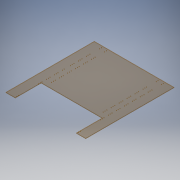
# Autodesk Inventor part: Top Aluminium Plate
Saved by Autodesk Inventor 2019.4 (Build 234330000, 330)
## iProperties
Created: 2019-12-08
Part Number: Top Aluminium Plate
Material: Polycarbonate, Smoke
Document SubType Name: Modeling
Designer: admin
Density: 1.2 g/cm^3
Appearance: Polycarbonate - Smoked
Mass: 1989.21 g
Surface Area: 8468.67 cm^2
Volume: 1657.67 cm^3
Author: admin
Autodesk Inventor part; units mm, degrees
ref_plane "YZ Plane" through (0, 0, 0) normal (1, 0, 0) x (0, 1, 0)
ref_plane "XZ Plane" through (0, 0, 0) normal (0, 1, 0) x (-1, 0, 0)
ref_plane "XY Plane" through (0, 0, 0) normal (0, 0, 1) x (1, 0, 0)
sketch "Sketch1" plane through (0, 0, 0) normal (0, 1, 0) x (-1, 0, 0)
  line L0 (323.8522, 485.9933) -> (327.8522, 485.9933) projected
  line L1 (327.8522, -234.0067) -> (327.8522, 485.9933) projected
  line L2 (-318.1478, -234.0067) -> (-322.1478, -234.0067) projected
  line L3 (-322.1478, -234.0067) -> (-322.1478, 485.9933) projected
  line L4 (327.8522, 485.9933) -> (-322.1478, 485.9933)
  line L5 (-322.1478, 485.9933) -> (-322.1478, -234.0067)
  line L6 (-322.1478, -234.0067) -> (327.8522, -234.0067)
  line L7 (327.8522, -234.0067) -> (327.8522, 485.9933)
  circle A0 centre (255.3522, -204.5067) radius 1.65 projected
  circle A1 centre (255.3522, -218.5067) radius 1.65 projected
  circle A2 centre (255.3522, 470.4933) radius 1.65 projected
  circle A3 centre (255.3522, 456.4933) radius 1.65 projected
  circle A4 centre (255.3522, 263.9913) radius 1.65 projected
  circle A5 centre (255.3522, 293.9913) radius 1.65 projected
  circle A6 centre (255.3522, 278.9913) radius 1.65 projected
  circle A7 centre (255.3522, -111.0087) radius 1.65 projected
  circle A8 centre (255.3522, -61.0087) radius 1.65 projected
  circle A9 centre (255.3522, -31.0087) radius 1.65 projected
  circle A10 centre (255.3522, 18.9913) radius 1.65 projected
  circle A11 centre (255.3522, 68.9913) radius 1.65 projected
  circle A12 centre (255.3522, 98.9913) radius 1.65 projected
  circle A13 centre (255.3522, 148.9913) radius 1.65 projected
  circle A14 centre (255.3522, 198.9913) radius 1.65 projected
  circle A15 centre (255.3522, 228.9913) radius 1.65 projected
  circle A16 centre (255.3522, 213.9913) radius 1.65 projected
  circle A17 centre (255.3522, 163.9913) radius 1.65 projected
  circle A18 centre (255.3522, 133.9913) radius 1.65 projected
  circle A19 centre (255.3522, 83.9913) radius 1.65 projected
  circle A20 centre (255.3522, 33.9913) radius 1.65 projected
  circle A21 centre (255.3522, 3.9913) radius 1.65 projected
  circle A22 centre (255.3522, -46.0087) radius 1.65 projected
  circle A23 centre (255.3522, -96.0087) radius 1.65 projected
  circle A24 centre (255.3522, -126.0087) radius 1.65 projected
  line L8 (251.8522, -234.0067) -> (251.8522, 485.9933) projected
  line L9 (251.8522, 485.9933) -> (258.8522, 485.9933) projected
  line L10 (258.8522, 485.9933) -> (258.8522, -234.0067) projected
  line L11 (258.8522, -234.0067) -> (251.8522, -234.0067) projected
  circle A25 centre (213.3522, -218.0067) radius 1.65 projected
  circle A26 centre (213.3522, -203.0067) radius 1.65 projected
  circle A27 centre (213.3522, 228.9913) radius 1.65 projected
  circle A28 centre (213.3522, 213.9913) radius 1.65 projected
  circle A29 centre (213.3522, 163.9913) radius 1.65 projected
  circle A30 centre (213.3522, 133.9913) radius 1.65 projected
  circle A31 centre (213.3522, 83.9913) radius 1.65 projected
  circle A32 centre (213.3522, 33.9913) radius 1.65 projected
  circle A33 centre (213.3522, 3.9913) radius 1.65 projected
  circle A34 centre (213.3522, -46.0087) radius 1.65 projected
  circle A35 centre (213.3522, -96.0087) radius 1.65 projected
  circle A36 centre (213.3522, -111.0087) radius 1.65 projected
  circle A37 centre (213.3522, -126.0087) radius 1.65 projected
  circle A38 centre (213.3522, -61.0087) radius 1.65 projected
  circle A39 centre (213.3522, -31.0087) radius 1.65 projected
  circle A40 centre (213.3522, 18.9913) radius 1.65 projected
  circle A41 centre (213.3522, 68.9913) radius 1.65 projected
  circle A42 centre (213.3522, 98.9913) radius 1.65 projected
  circle A43 centre (213.3522, 148.9913) radius 1.65 projected
  circle A44 centre (213.3522, 198.9913) radius 1.65 projected
  line L12 (209.8522, 274.709) -> (216.8522, 274.709) projected
  line L13 (216.8522, -234.0067) -> (216.8522, 274.709) projected
  line L14 (216.8522, -234.0067) -> (209.8522, -234.0067) projected
  line L15 (209.8522, -234.0067) -> (209.8522, 274.709) projected
  circle A45 centre (-249.6478, -204.5067) radius 1.65 projected
  circle A46 centre (-249.6478, -218.5067) radius 1.65 projected
  circle A47 centre (-249.6478, 470.4933) radius 1.65 projected
  circle A48 centre (-249.6478, 456.4933) radius 1.65 projected
  circle A49 centre (-249.6478, 263.9913) radius 1.65 projected
  circle A50 centre (-249.6478, 293.9913) radius 1.65 projected
  circle A51 centre (-249.6478, 278.9913) radius 1.65 projected
  circle A52 centre (-249.6478, -111.0087) radius 1.65 projected
  circle A53 centre (-249.6478, -61.0087) radius 1.65 projected
  circle A54 centre (-249.6478, -31.0087) radius 1.65 projected
  circle A55 centre (-249.6478, 18.9913) radius 1.65 projected
  circle A56 centre (-249.6478, 68.9913) radius 1.65 projected
  circle A57 centre (-249.6478, 98.9913) radius 1.65 projected
  circle A58 centre (-249.6478, 148.9913) radius 1.65 projected
  circle A59 centre (-249.6478, 198.9913) radius 1.65 projected
  circle A60 centre (-249.6478, 228.9913) radius 1.65 projected
  circle A61 centre (-249.6478, 213.9913) radius 1.65 projected
  circle A62 centre (-249.6478, 163.9913) radius 1.65 projected
  circle A63 centre (-249.6478, 133.9913) radius 1.65 projected
  circle A64 centre (-249.6478, 83.9913) radius 1.65 projected
  circle A65 centre (-249.6478, 33.9913) radius 1.65 projected
  circle A66 centre (-249.6478, 3.9913) radius 1.65 projected
  circle A67 centre (-249.6478, -46.0087) radius 1.65 projected
  circle A68 centre (-249.6478, -96.0087) radius 1.65 projected
  circle A69 centre (-249.6478, -126.0087) radius 1.65 projected
  line L16 (-246.1478, -234.0067) -> (-246.1478, 485.9933) projected
  line L17 (-253.1478, -234.0067) -> (-246.1478, -234.0067) projected
  line L18 (-253.1478, 485.9933) -> (-253.1478, -234.0067) projected
  line L19 (-246.1478, 485.9933) -> (-253.1478, 485.9933) projected
  circle A70 centre (-207.6478, -218.0067) radius 1.65 projected
  circle A71 centre (-207.6478, -203.0067) radius 1.65 projected
  circle A72 centre (-207.6478, 228.9913) radius 1.65 projected
  circle A73 centre (-207.6478, 213.9913) radius 1.65 projected
  circle A74 centre (-207.6478, 163.9913) radius 1.65 projected
  circle A75 centre (-207.6478, 133.9913) radius 1.65 projected
  circle A76 centre (-207.6478, 83.9913) radius 1.65 projected
  circle A77 centre (-207.6478, 33.9913) radius 1.65 projected
  circle A78 centre (-207.6478, 3.9913) radius 1.65 projected
  circle A79 centre (-207.6478, -46.0087) radius 1.65 projected
  circle A80 centre (-207.6478, -96.0087) radius 1.65 projected
  circle A81 centre (-207.6478, -111.0087) radius 1.65 projected
  circle A82 centre (-207.6478, -126.0087) radius 1.65 projected
  circle A83 centre (-207.6478, -61.0087) radius 1.65 projected
  circle A84 centre (-207.6478, -31.0087) radius 1.65 projected
  circle A85 centre (-207.6478, 18.9913) radius 1.65 projected
  circle A86 centre (-207.6478, 68.9913) radius 1.65 projected
  circle A87 centre (-207.6478, 98.9913) radius 1.65 projected
  circle A88 centre (-207.6478, 148.9913) radius 1.65 projected
  circle A89 centre (-207.6478, 198.9913) radius 1.65 projected
  line L20 (-204.1478, 274.709) -> (-211.1478, 274.709) projected
  line L21 (-204.1478, -234.0067) -> (-204.1478, 274.709) projected
  line L22 (-211.1478, -234.0067) -> (-204.1478, -234.0067) projected
  line L23 (-211.1478, -234.0067) -> (-211.1478, 274.709) projected
  constraints: 6 end point, 2 horizontal, 1 parallel, 1 perpendicular, 3 other
extrude "Extrusion1" add sketch "Sketch1" along normal blind 4 contours L0 L1 L6 L10 L4 | L10 L6 L8 L4 | L8 L6 L13 L12 L15 L21 L20 L23 L16 L4 | L16 L6 L18 L4 | L18 L6 L2 L3 L4 | L6 L15 L12 L13 | L23 L20 L21 L6 | A0 | A1 | A2 | A3 | A4 | A5 | A6 | A7 | A8 | A9 | A10 | A11 | A12 | A13 | A14 | A15 | A16 | A17 | A18 | A19 | A20 | A21 | A22 | A23 | A24 | A25 | A26 | A27 | A28 | A29 | A30 | A31 | A32 | A33 | A34 | A35 | A36 | A37 | A38 | A39 | A40 | A41 | A42 | A43 | A44 | A45 | A46 | A47 | A48 | A49 | A50 | A51 | A52 | A53 | A54 | A55 | A56 | A57 | A58 | A59 | A60 | A61 | A62 | A63 | A64 | A65 | A66 | A67 | A68 | A69 | A70 | A71 | A72 | A73 | A74 | A75 | A76 | A77 | A78 | A79 | A80 | A81 | A82 | A83 | A84 | A85 | A86 | A87 | A88 | A89
sketch "Sketch2" plane through (0, 0, 0) normal (0, -1, 0) x (1, 0, 0)
  circle A0 centre (-255.3522, -204.5067) radius 1.65 projected
  circle A1 centre (-255.3522, -218.5067) radius 1.65 projected
  circle A2 centre (-255.3522, 470.4933) radius 1.65 projected
  circle A3 centre (-255.3522, 456.4933) radius 1.65 projected
  circle A4 centre (-255.3522, 263.9913) radius 1.65 projected
  circle A5 centre (-255.3522, 293.9913) radius 1.65 projected
  circle A6 centre (-255.3522, 278.9913) radius 1.65 projected
  circle A7 centre (-255.3522, -111.0087) radius 1.65 projected
  circle A8 centre (-255.3522, -61.0087) radius 1.65 projected
  circle A9 centre (-255.3522, -31.0087) radius 1.65 projected
  circle A10 centre (-255.3522, 18.9913) radius 1.65 projected
  circle A11 centre (-255.3522, 68.9913) radius 1.65 projected
  circle A12 centre (-255.3522, 98.9913) radius 1.65 projected
  circle A13 centre (-255.3522, 148.9913) radius 1.65 projected
  circle A14 centre (-255.3522, 198.9913) radius 1.65 projected
  circle A15 centre (-255.3522, 228.9913) radius 1.65 projected
  circle A16 centre (-255.3522, 213.9913) radius 1.65 projected
  circle A17 centre (-255.3522, 163.9913) radius 1.65 projected
  circle A18 centre (-255.3522, 133.9913) radius 1.65 projected
  circle A19 centre (-255.3522, 83.9913) radius 1.65 projected
  circle A20 centre (-255.3522, 33.9913) radius 1.65 projected
  circle A21 centre (-255.3522, 3.9913) radius 1.65 projected
  circle A22 centre (-255.3522, -46.0087) radius 1.65 projected
  circle A23 centre (-255.3522, -96.0087) radius 1.65 projected
  circle A24 centre (-255.3522, -126.0087) radius 1.65 projected
  line L0 (-251.8522, -234.0067) -> (-251.8522, 485.9933) projected
  line L1 (-251.8522, 485.9933) -> (-258.8522, 485.9933) projected
  line L2 (-258.8522, 485.9933) -> (-258.8522, -234.0067) projected
  line L3 (-258.8522, -234.0067) -> (-251.8522, -234.0067) projected
  circle A25 centre (-213.3522, -218.0067) radius 1.65 projected
  circle A26 centre (-213.3522, -203.0067) radius 1.65 projected
  circle A27 centre (-213.3522, 228.9913) radius 1.65 projected
  circle A28 centre (-213.3522, 213.9913) radius 1.65 projected
  circle A29 centre (-213.3522, 163.9913) radius 1.65 projected
  circle A30 centre (-213.3522, 133.9913) radius 1.65 projected
  circle A31 centre (-213.3522, 83.9913) radius 1.65 projected
  circle A32 centre (-213.3522, 33.9913) radius 1.65 projected
  circle A33 centre (-213.3522, 3.9913) radius 1.65 projected
  circle A34 centre (-213.3522, -46.0087) radius 1.65 projected
  circle A35 centre (-213.3522, -96.0087) radius 1.65 projected
  circle A36 centre (-213.3522, -111.0087) radius 1.65 projected
  circle A37 centre (-213.3522, -126.0087) radius 1.65 projected
  circle A38 centre (-213.3522, -61.0087) radius 1.65 projected
  circle A39 centre (-213.3522, -31.0087) radius 1.65 projected
  circle A40 centre (-213.3522, 18.9913) radius 1.65 projected
  circle A41 centre (-213.3522, 68.9913) radius 1.65 projected
  circle A42 centre (-213.3522, 98.9913) radius 1.65 projected
  circle A43 centre (-213.3522, 148.9913) radius 1.65 projected
  circle A44 centre (-213.3522, 198.9913) radius 1.65 projected
  line L4 (-209.8522, 274.709) -> (-216.8522, 274.709) projected
  line L5 (-216.8522, -234.0067) -> (-216.8522, 274.709) projected
  line L6 (-216.8522, -234.0067) -> (-209.8522, -234.0067) projected
  line L7 (-209.8522, -234.0067) -> (-209.8522, 274.709) projected
  circle A45 centre (249.6478, -204.5067) radius 1.65 projected
  circle A46 centre (249.6478, -218.5067) radius 1.65 projected
  circle A47 centre (249.6478, 470.4933) radius 1.65 projected
  circle A48 centre (249.6478, 456.4933) radius 1.65 projected
  circle A49 centre (249.6478, 263.9913) radius 1.65 projected
  circle A50 centre (249.6478, 293.9913) radius 1.65 projected
  circle A51 centre (249.6478, 278.9913) radius 1.65 projected
  circle A52 centre (249.6478, -111.0087) radius 1.65 projected
  circle A53 centre (249.6478, -61.0087) radius 1.65 projected
  circle A54 centre (249.6478, -31.0087) radius 1.65 projected
  circle A55 centre (249.6478, 18.9913) radius 1.65 projected
  circle A56 centre (249.6478, 68.9913) radius 1.65 projected
  circle A57 centre (249.6478, 98.9913) radius 1.65 projected
  circle A58 centre (249.6478, 148.9913) radius 1.65 projected
  circle A59 centre (249.6478, 198.9913) radius 1.65 projected
  circle A60 centre (249.6478, 228.9913) radius 1.65 projected
  circle A61 centre (249.6478, 213.9913) radius 1.65 projected
  circle A62 centre (249.6478, 163.9913) radius 1.65 projected
  circle A63 centre (249.6478, 133.9913) radius 1.65 projected
  circle A64 centre (249.6478, 83.9913) radius 1.65 projected
  circle A65 centre (249.6478, 33.9913) radius 1.65 projected
  circle A66 centre (249.6478, 3.9913) radius 1.65 projected
  circle A67 centre (249.6478, -46.0087) radius 1.65 projected
  circle A68 centre (249.6478, -96.0087) radius 1.65 projected
  circle A69 centre (249.6478, -126.0087) radius 1.65 projected
  line L8 (246.1478, -234.0067) -> (246.1478, 485.9933) projected
  line L9 (253.1478, -234.0067) -> (246.1478, -234.0067) projected
  line L10 (253.1478, 485.9933) -> (253.1478, -234.0067) projected
  line L11 (246.1478, 485.9933) -> (253.1478, 485.9933) projected
  circle A70 centre (207.6478, -218.0067) radius 1.65 projected
  circle A71 centre (207.6478, -203.0067) radius 1.65 projected
  circle A72 centre (207.6478, 228.9913) radius 1.65 projected
  circle A73 centre (207.6478, 213.9913) radius 1.65 projected
  circle A74 centre (207.6478, 163.9913) radius 1.65 projected
  circle A75 centre (207.6478, 133.9913) radius 1.65 projected
  circle A76 centre (207.6478, 83.9913) radius 1.65 projected
  circle A77 centre (207.6478, 33.9913) radius 1.65 projected
  circle A78 centre (207.6478, 3.9913) radius 1.65 projected
  circle A79 centre (207.6478, -46.0087) radius 1.65 projected
  circle A80 centre (207.6478, -96.0087) radius 1.65 projected
  circle A81 centre (207.6478, -111.0087) radius 1.65 projected
  circle A82 centre (207.6478, -126.0087) radius 1.65 projected
  circle A83 centre (207.6478, -61.0087) radius 1.65 projected
  circle A84 centre (207.6478, -31.0087) radius 1.65 projected
  circle A85 centre (207.6478, 18.9913) radius 1.65 projected
  circle A86 centre (207.6478, 68.9913) radius 1.65 projected
  circle A87 centre (207.6478, 98.9913) radius 1.65 projected
  circle A88 centre (207.6478, 148.9913) radius 1.65 projected
  circle A89 centre (207.6478, 198.9913) radius 1.65 projected
  line L12 (204.1478, 274.709) -> (211.1478, 274.709) projected
  line L13 (204.1478, -234.0067) -> (204.1478, 274.709) projected
  line L14 (211.1478, -234.0067) -> (204.1478, -234.0067) projected
  line L15 (211.1478, -234.0067) -> (211.1478, 274.709) projected
  line L16 (-251.8522, 485.9933) -> (-126.8522, 485.9933)
  line L17 (-126.8522, 485.9933) -> (-126.8522, 274.709) construction
  line L18 (-126.8522, 274.709) -> (-251.8522, 274.709)
  line L19 (-251.8522, 274.709) -> (-251.8522, 485.9933)
  line L20 (246.1478, 485.9933) -> (121.1478, 485.9933)
  line L21 (121.1478, 485.9933) -> (121.1478, 274.709) construction
  line L22 (121.1478, 274.709) -> (246.1478, 274.709)
  line L23 (246.1478, 274.709) -> (246.1478, 485.9933)
  line L24 (121.1478, 274.709) -> (-126.8522, 274.709)
  line L25 (-126.8522, 485.9933) -> (121.1478, 485.9933)
  point P0 (0, 0)
  dimension "d2" = 125
  dimension "d3" = 125
  constraints: 20 end point, 5 parallel, 3 horizontal, 2 collinear, 2 perpendicular
  measures "d2" distance of L17.end L18.end
  measures "d3" distance of L21.end L22.end
extrude "Extrusion2" cut sketch "Sketch2" against normal through all contours A0 | A1 | A2 | A3 | A4 | A5 | A6 | A7 | A8 | A9 | A10 | A12 | A13 | A14 | A15 | A16 | A17 | A18 | A19 | A20 | A21 | A22 | A23 | A24 | L0 L16 L25 L20 L8 L22 L12 L24 L18 L4 | A25 | A26 | A27 | A28 | A29 | A30 | A31 | A32 | A33 | A34 | A35 | A36 | A37 | A38 | A39 | A40 | A41 | A42 | A43 | A44 | A45 | A46 | A47 | A48 | A49 | A50 | A51 | A52 | A53 | A54 | A55 | A56 | A57 | A58 | A59 | A60 | A61 | A62 | A63 | A64 | A65 | A66 | A67 | A68 | A69 | A70 | A71 | A72 | A73 | A74 | A75 | A76 | A77 | A78 | A79 | A80 | A81 | A82 | A83 | A84 | A85 | A86 | A87 | A88 | A89
body "Solid1"
